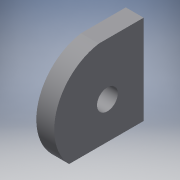
# Autodesk Inventor part: weight_holder_string_loop
Saved by Autodesk Inventor 2016 (Build 200138000, 138)
## iProperties
Created: 2016-08-02
Part Number: weight_holder_string_loop
Material: Generic
Document SubType Name: Modeling
Designer: ajar021
Density: 1 g/cm^3
Appearance: Default
Author: ajar021
Autodesk Inventor part; units mm, degrees
ref_plane "YZ Plane" through (0, 0, 0) normal (1, 0, 0) x (0, 1, 0)
ref_plane "XZ Plane" through (0, 0, 0) normal (0, 1, 0) x (-1, 0, 0)
ref_plane "XY Plane" through (0, 0, 0) normal (0, 0, 1) x (1, 0, 0)
sketch "Sketch1" plane through (0, 0, 0) normal (0, 0, 1) x (1, 0, 0)
  line L0 (7.5, 7.5) -> (-7.5, 7.5) projected
  line L1 (-7.5, -7.5) -> (7.5, -7.5) projected
  line L2 (-1.5, 7.5) -> (1.5, 7.5)
  line L3 (1.5, 7.5) -> (1.5, -7.5)
  line L4 (1.5, -7.5) -> (-1.5, -7.5)
  line L5 (-1.5, -7.5) -> (-1.5, 7.5)
  line L6 (-1.5, 7.5) -> (1.5, -7.5) construction
  line L7 (1.5, 7.5) -> (-1.5, -7.5) construction
  point P0 (0, 0)
  dimension "d0" = 3
  constraints: 12 end point, 2 midpoint, 2 parallel, 1 horizontal, 1 perpendicular, 1 point on line
  measures "d0" distance of L2.end L2.start
extrude "Extrusion1" add sketch "Sketch1" along normal blind 15
sketch "Sketch2" plane through (1.5, -7.5, 0) normal (1, 0, 0) x (0, 0, -1)
  line L0 (0, 15) -> (0, 0) projected
  line L1 (0, 15) -> (-15, 15) projected
  line L2 (-15, 0) -> (-15, 15) projected
  line L3 (-15, 15) -> (-7.5, 15)
  line L4 (0, 15) -> (-15, 15) projected
  line L5 (0, 0) -> (-15, 0) projected
  line L6 (0, 0) -> (-15, 0) projected
  arc A0 (-7.5, 15) -> (-7.5, 0) centre (-7.5, 7.5) ccw
  line L7 (-15, 15) -> (-15, 0) projected
  circle A1 centre (-7.5, 7.5) radius 1.75
  point P0 (0, 7.5)
  point P1 (-10, 7.5)
  dimension "d3" = 7.5
  dimension "d7" = 3.5
  constraints: 2 centre point, 2 end point, 2 midpoint, 2 point on circle, 1 coincident, 1 tangent
  measures "d3" distance of L1.end L3.end
  measures "d7" diameter of A1
extrude "Extrusion2" cut sketch "Sketch2" against normal up to next contours A0 L2 L1 | L5 L2 A0 | A1
body "Solid1"
